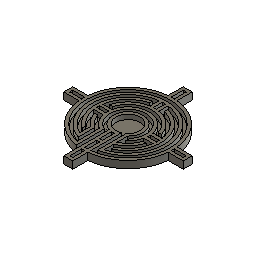
Labyrinth1 (5-gängig) v1 (Autodesk Fusion 360 design; units mm, degrees)
Autodesk Fusion 360 part; units mm, degrees
sketch "Skizze1" plane through (0, 0, 0) normal (0, 1, 0) x (1, 0, 0)
  circle A0 centre (0, 0) radius 15 construction
  circle A1 centre (0, 0) radius 20 construction
  circle A2 centre (0, 0) radius 25 construction
  circle A3 centre (0, 0) radius 30 construction
  circle A4 centre (0, 0) radius 35 construction
  line L0 (0, 0) -> (0, 68.1169) construction
  line L1 (0, 0) -> (0, -68.6498) construction
  line L2 (-1.25, 0) -> (-1.25, 68.1169) construction
  line L3 (-1.25, 0) -> (-1.25, -68.6498) construction
  line L4 (1.25, 0) -> (1.25, 68.1169) construction
  line L5 (1.25, 0) -> (1.25, -68.6498) construction
  line L6 (-3.75, 0) -> (-3.75, 68.1169) construction
  line L7 (-3.75, 0) -> (-3.75, -68.6498) construction
  line L8 (3.75, 0) -> (3.75, 68.1169) construction
  line L9 (3.75, 0) -> (3.75, -68.6498) construction
  line L10 (-6.25, 0) -> (-6.25, -68.6498) construction
  line L11 (-6.25, 0) -> (-6.25, 68.1169) construction
  line L12 (6.25, 0) -> (6.25, 68.1169) construction
  line L13 (6.25, 0) -> (6.25, -68.6498) construction
  line L14 (0, 0) -> (75.7523, 0) construction
  line L15 (0, 0) -> (-77.2035, 0) construction
  line L16 (0, -1.25) -> (-77.2035, -1.25) construction
  line L17 (0, -1.25) -> (75.7523, -1.25) construction
  line L18 (0, 1.25) -> (75.7523, 1.25) construction
  line L19 (0, 1.25) -> (-77.2035, 1.25) construction
  line L20 (0, 3.75) -> (75.7523, 3.75) construction
  line L21 (0, -3.75) -> (-77.2035, -3.75) construction
  line L22 (0, -3.75) -> (75.7523, -3.75) construction
  line L23 (0, -6.25) -> (75.7523, -6.25) construction
  line L24 (0, -6.25) -> (-77.2035, -6.25) construction
  line L25 (0, 6.25) -> (-77.2035, 6.25) construction
  line L26 (0, 6.25) -> (75.7523, 6.25) construction
  line L27 (0, 0) -> (50, 0) construction
  line L28 (0, 0) -> (-50, 0) construction
  line L29 (0, 0) -> (0, 50) construction
  line L30 (0, 0) -> (0, -50) construction
  line L31 (0, 50) -> (3.75, 50) construction
  line L32 (-50, 0) -> (-50, 3.75) construction
  line L33 (-50, 3.75) -> (50, 3.75) construction
  line L34 (50, 3.75) -> (50, -3.75) construction
  line L35 (50, -3.75) -> (-50, -3.75) construction
  line L36 (-50, -3.75) -> (-50, 3.75) construction
  line L37 (50, 3.75) -> (50, -3.75)
  line L38 (-50, -3.75) -> (-50, 3.75)
  line L39 (3.75, 50) -> (-3.75, 50)
  line L40 (-3.75, -50) -> (3.75, -50)
  circle A5 centre (0, 0) radius 12.5 construction
  arc A6 (6.25, -7.8334) -> (3.75, -9.2931) centre (0, 0) ccw
  line L41 (-6.25, -44.5639) -> (-6.25, -13.6359)
  line L42 (-6.25, 39.5087) -> (-6.25, 42.0379)
  circle A7 centre (0, 0) radius 37.5
  line L43 (-8.75, 0) -> (-8.75, -50) construction
  line L44 (-11.25, 0) -> (-11.25, -50) construction
  line L45 (11.25, 0) -> (11.25, -50) construction
  line L46 (8.75, 0) -> (8.75, -68.6498) construction
  line L47 (-1.25, -12.4373) -> (-1.25, -44.9826)
  line L48 (1.25, -12.4373) -> (1.25, -44.9826)
  arc A8 (-1.25, -12.4373) -> (1.25, -12.4373) centre (0, 0) ccw
  line L49 (3.75, -9.2931) -> (3.75, -42.3342)
  arc A9 (8.75, -8.9268) -> (-3.75, -11.9242) centre (0, 0) ccw
  line L50 (8.75, -39.0312) -> (8.7506, -41.5894)
  line L51 (-6.25, -44.5639) -> (-6.25, -49.6078)
  arc A10 (11.25, -9.9216) -> (-6.25, -13.6359) centre (0, 0) ccw
  arc A11 (11.25, -13.4048) -> (17.0935, -3.75) centre (0, 0) ccw
  arc A12 (8.75, -17.9844) -> (18.9984, -6.25) centre (0, 0) ccw
  line L52 (11.25, -9.9216) -> (11.25, -13.4048)
  arc A13 (8.75, -20.7289) -> (21.6145, -6.25) centre (0, 0) ccw
  line L53 (18.9984, -6.25) -> (21.6145, -6.25)
  arc A14 (11.25, -22.4692) -> (24.8468, -3.75) centre (0, 0) ccw
  arc A15 (11.25, -25.0936) -> (27.2431, -3.75) centre (0, 0) ccw
  line L54 (11.25, -22.4692) -> (11.25, -25.0936)
  arc A16 (27.2431, -3.75) -> (27.2431, 3.75) centre (0, 0) ccw
  arc A17 (27.2431, 3.75) -> (6.25, 26.7804) centre (0, 0) ccw
  arc A18 (24.7171, 3.75) -> (6.25, 24.2061) centre (0, 0) ccw
  line L55 (6.25, 26.7804) -> (6.25, 24.2061)
  arc A19 (8.75, -28.6956) -> (3.75, 29.7647) centre (0, 0) ccw
  arc A20 (6.25, -31.8934) -> (-11.25, -30.4908) centre (0, 0) ccw
  arc A21 (3.75, -34.7985) -> (-8.75, -33.8886) centre (0, 0) ccw
  arc A22 (17.0935, 3.75) -> (-8.75, -15.1554) centre (0, 0) ccw
  line L56 (-8.75, -15.1554) -> (-8.75, -33.8886)
  arc A23 (18.9984, 6.25) -> (3.75, 19.6453) centre (0, 0) ccw
  line L57 (3.75, 29.7647) -> (3.75, 19.6453)
  arc A24 (21.6145, 6.25) -> (3.75, 22.1853) centre (0, 0) ccw
  line L58 (18.9984, 6.25) -> (21.6145, 6.25)
  line L59 (3.75, 29.7647) -> (3.75, 32.2829)
  line L60 (-3.75, -11.9242) -> (-3.75, -50)
  arc A25 (3.75, -37.312) -> (-6.25, -36.9755) centre (0, 0) ccw
  line L61 (37.2821, 3.75) -> (50, 3.75)
  line L62 (50, 3.75) -> (50, -3.75)
  line L63 (50, -3.75) -> (37.312, -3.75)
  line L64 (-37.312, 3.75) -> (-50, 3.75)
  line L65 (-50, -3.75) -> (-37.312, -3.75)
  line L66 (-3.879, 37.2988) -> (-3.75, 50)
  line L67 (3.75, 50) -> (3.6612, 37.3208)
  arc A26 (3.75, 19.6453) -> (-18.9984, 6.25) centre (0, 0) ccw
  line L68 (6.25, -31.8934) -> (6.25, -7.8334)
  line L69 (8.75, -28.6956) -> (8.75, -20.7289)
  line L70 (8.75, -17.9844) -> (8.75, -8.9268)
  line L71 (-3.75, 32.2829) -> (-3.75, 19.6453)
  arc A27 (1.25, 22.4653) -> (-1.25, 22.4653) centre (0, 0) ccw
  arc A28 (1.25, 29.9739) -> (-1.25, 29.9739) centre (0, 0) ccw
  line L72 (1.25, 22.4653) -> (1.25, 29.9739)
  line L73 (-1.25, 22.4653) -> (-1.25, 29.9739)
  line L74 (17.0935, 3.75) -> (24.7171, 3.75)
  line L75 (17.0935, -3.75) -> (24.8468, -3.75)
  line L76 (3.75, -37.312) -> (3.75, -50)
  line L77 (-11.25, -16.5359) -> (-11.25, -30.4908)
  line L78 (-16.25, -16.5359) -> (-16.25, -30.4908) construction
  line L79 (-13.75, -16.5359) -> (-13.75, -30.4908) construction
  arc A29 (-18.9984, -6.25) -> (-11.25, -16.5359) centre (0, 0) ccw
  arc A30 (-21.6145, -6.25) -> (-13.75, -17.8098) centre (0, 0) ccw
  arc A31 (-6.25, 29.3417) -> (-13.75, -26.6634) centre (0, 0) ccw
  arc A32 (-6.25, 26.7804) -> (-26.7804, 6.25) centre (0, 0) ccw
  arc A33 (-3.75, 29.7647) -> (-6.25, 29.3417) centre (0, 0) ccw
  line L80 (-18.9984, -6.25) -> (-21.6145, -6.25)
  line L81 (-13.75, -17.8098) -> (-13.75, -26.6634)
  arc A34 (-26.7804, 6.25) -> (-16.25, -22.1853) centre (0, 0) ccw
  arc A35 (-6.25, 24.2061) -> (-24.7171, 3.75) centre (0, 0) ccw
  line L82 (-6.25, 26.7804) -> (-6.25, 24.2061)
  line L83 (-24.7171, 3.75) -> (-27.2431, 3.75)
  arc A36 (-24.791, -3.75) -> (-16.25, -19.0943) centre (0, 0) ccw
  line L84 (-16.25, -19.0943) -> (-16.25, -22.1853)
  line L85 (-24.791, -3.75) -> (-27.2431, -3.75)
  line L86 (-27.2431, 3.75) -> (-17.0935, 3.75)
  line L87 (-27.2431, -3.75) -> (-17.051, -3.75)
  arc A37 (-3.75, 22.1853) -> (-21.6145, 6.25) centre (0, 0) ccw
  line L88 (-21.6145, 6.25) -> (-18.9984, 6.25)
  line L89 (3.75, 47.5) -> (-3.75, 47.5) construction
  line L90 (-1.25, 47.5) -> (1.25, 47.5)
  line L91 (1.25, 47.5) -> (1.2613, 37.4788)
  line L92 (-1.299, 37.4775) -> (-1.25, 47.5)
  line L93 (-47.4997, -3.75) -> (-47.4997, 3.75) construction
  line L94 (47.4997, 3.75) -> (47.4997, -3.75) construction
  line L95 (-47.4997, -1.25) -> (-37.4792, -1.25)
  line L96 (-47.4997, 1.25) -> (-47.4997, -1.25)
  line L97 (-47.4997, 1.25) -> (-37.4792, 1.25)
  line L98 (47.4997, 1.25) -> (37.4792, 1.25)
  line L99 (47.4997, -1.25) -> (37.4792, -1.25)
  line L100 (47.4997, 1.25) -> (47.4997, -1.25)
  arc A38 (-24.9687, 1.25) -> (-24.9687, -1.25) centre (0, 0) ccw
  arc A39 (17.4553, -1.25) -> (17.4553, 1.25) centre (0, 0) ccw
  arc A40 (24.9687, -1.25) -> (24.9687, 1.25) centre (0, 0) ccw
  line L101 (17.4553, 1.25) -> (24.9687, 1.25)
  line L102 (17.4553, -1.25) -> (24.9687, -1.25)
  line L103 (-24.9687, 1.25) -> (-17.4553, 1.25)
  line L104 (-24.9687, -1.25) -> (-17.4553, -1.25)
  arc A41 (-1.25, -47.4835) -> (1.25, -47.4835) centre (0, 0) ccw
  line L105 (1.25, -37.4792) -> (1.25, -47.4835)
  line L106 (-1.25, -37.4567) -> (-1.25, -47.4835)
  arc A42 (-1.25, -24.9687) -> (1.25, -24.9687) centre (0, 0) ccw
  arc A43 (-1.25, -22.4653) -> (1.25, -22.4653) centre (0, 0) ccw
  arc A44 (-1.25, -34.8756) -> (1.25, -34.8756) centre (0, 0) ccw
  dimension "d9" = 1.25
  dimension "d10" = -1.25
  dimension "d11" = 3.75
  dimension "d12" = -3.75
  dimension "d13" = 6.25
  dimension "d15" = -6.25
  dimension "d16" = 1.25
  dimension "d17" = -1.25
  dimension "d19" = -3.75
  dimension "d20" = 6.25
  dimension "d21" = -6.25
  dimension "d22" = 50
  dimension "d23" = 50
  dimension "d24" = 50
  dimension "d25" = 50
  dimension "d44" = 37.5
  dimension "d46" = 5
  dimension "d47" = 2.5
  dimension "d48" = 22.5
  dimension "d50" = 22.5
  dimension "d51" = -2.5
  dimension "d52" = 2.5003
  dimension "d53" = 2.5003
  dimension "d54" = 17.5
  dimension "d59" = 47.5
  constraint coincident A0.centre A1.centre
  constraint concentric A0 A1
  constraint concentric A3 A4
  constraint vertical L0
  constraint vertical L1
  constraint horizontal L14
  constraint horizontal L15
  constraint parallel L14 L27
  constraint parallel L16 L28
  constraint parallel L0 L29
  constraint parallel L1 L30
  constraint coincident L8 L31.end
  constraint perpendicular L8 L31
  constraint horizontal L33
  constraint vertical L34
  constraint horizontal L35
  constraint vertical L36
  constraint coincident L22 L34.end
  constraint vertical L37
  constraint vertical L38
  constraint horizontal L39
  constraint horizontal L40
  constraint coincident L7 L40.start
  constraint concentric A1 A5
  constraint coincident L13 A6.start
  constraint coincident L9 A6.end
  constraint coincident L10 L41.start
  constraint coincident L10 L41.end
  constraint coincident A0 L41.end
  constraint coincident L11 L42.start
  constraint coincident L11 L42.end
  constraint coincident L3 L47.start
  constraint coincident A5 L47.start
  constraint coincident L3 L47.end
  constraint coincident A5 L48.start
  constraint coincident L5 L48.start
  constraint coincident L5 L48.end
  constraint coincident L9 L49.end
  constraint coincident L7 A9.end
  constraint coincident A5 A9.start
  constraint coincident L46 A9.start
  constraint coincident L46 L50.start
  constraint coincident L10 L51.end
  constraint coincident L45 A10.start
  constraint coincident L22 A11.end
  constraint coincident L45 A11.start
  constraint coincident L23 A12.end
  constraint coincident A1 A12.start
  constraint coincident L46 A13.start
  constraint coincident L23 A13.end
  constraint coincident L45 A14.start
  constraint coincident L22 A14.end
  constraint coincident L45 A15.start
  constraint coincident L22 A15.end
  constraint coincident L12 A17.end
  constraint coincident L20 A18.start
  constraint coincident L12 A18.end
  constraint coincident A2 A18.end
  constraint coincident L8 A19.end
  constraint coincident L46 A19.start
  constraint coincident L44 A20.end
  constraint coincident L43 A21.end
  constraint coincident A4 A21.start
  constraint coincident L9 A21.start
  constraint coincident L20 A22.start
  constraint coincident L43 A22.end
  constraint coincident L8 A23.end
  constraint coincident L26 A23.start
  constraint coincident A1 A23.start
  constraint coincident L8 A24.end
  constraint coincident L26 A24.start
  constraint coincident L8 L59.end
  constraint coincident A20 L59.end
  constraint coincident L10 A25.end
  constraint coincident L33 L61.start
  constraint perpendicular L34 L61
  constraint coincident L35 L63.end
  constraint coincident A7 L63.end
  constraint coincident L33 L64.start
  constraint coincident A7 L64.start
  constraint perpendicular L32 L64
  constraint coincident L21 L65.end
  constraint coincident A7 L65.end
  constraint coincident A7 L66.start
  constraint coincident A25 L66.start
  constraint coincident A25 L67.end
  constraint coincident A7 L67.end
  constraint coincident L25 A26.end
  constraint parallel L13 L68
  constraint parallel L46 L70
  constraint coincident L6 L71.start
  constraint coincident A20 L71.start
  constraint coincident L6 L71.end
  constraint coincident A26 L71.end
  constraint coincident A1 L71.end
  constraint coincident L2 A27.end
  constraint coincident L4 A27.start
  constraint coincident L2 A28.end
  constraint coincident A3 A28.start
  constraint coincident L4 A28.start
  constraint perpendicular L40 L76
  constraint coincident A1 L77.start
  constraint coincident L44 L77.start
  constraint coincident L24 A29.start
  constraint coincident L79 A30.end
  constraint coincident L24 A30.start
  constraint coincident L11 A31.start
  constraint coincident L79 A31.end
  constraint coincident A3 A31.end
  constraint coincident L25 A32.end
  constraint coincident L11 A32.start
  constraint coincident L6 A33.start
  constraint coincident L78 A34.end
  constraint coincident L35 A36.start
  constraint coincident L33 A35.end
  constraint coincident A2 A35.end
  constraint coincident L11 A35.start
  constraint coincident L33 L83.end
  constraint coincident A34 L83.end
  constraint coincident L78 A36.end
  constraint coincident L21 L85.end
  constraint coincident A34 L85.end
  constraint coincident L33 L86.end
  constraint coincident A22 L86.end
  constraint coincident L21 L87.end
  constraint coincident L25 A37.end
  constraint coincident L6 A37.start
  constraint coincident L89 L90.start
  constraint coincident L2 L90.start
  constraint coincident L4 L90.end
  constraint coincident L89 L90.end
  constraint midpoint A25 L91.end
  constraint coincident A7 L92.start
  constraint coincident A25 L92.start
  constraint coincident L19 L96.start
  constraint coincident L93 L96.start
  constraint coincident L16 L95.start
  constraint coincident L93 L95.start
  constraint coincident L16 L95.end
  constraint coincident A7 L95.end
  constraint coincident A25 L95.end
  constraint coincident L19 L97.end
  constraint coincident A25 L97.end
  constraint coincident A7 L97.end
  constraint coincident L94 L98.start
  constraint coincident L18 L98.start
  constraint coincident A7 L98.end
  constraint coincident L18 L98.end
  constraint coincident A25 L98.end
  constraint coincident L94 L99.start
  constraint coincident L17 L99.start
  constraint coincident L17 L99.end
  constraint coincident A7 L99.end
  constraint coincident L16 A38.end
  constraint coincident L19 A38.start
  constraint coincident A2 A38.start
  constraint coincident L18 A39.end
  constraint coincident L17 A39.start
  constraint coincident L17 A40.start
  constraint coincident L18 A40.end
  constraint coincident A2 A40.end
  constraint coincident L19 L103.end
  constraint coincident A22 L103.end
  constraint coincident A22 L104.end
  constraint coincident L16 L104.end
  constraint coincident L3 A41.start
  constraint coincident L5 A41.end
  constraint coincident L48 L105.start
  constraint coincident A7 L105.start
  constraint coincident L47 L106.start
  constraint coincident L3 A42.start
  constraint coincident A2 A42.end
  constraint coincident L48 A42.end
  constraint coincident L3 A43.start
  constraint coincident L48 A43.end
  constraint coincident L3 A44.start
  constraint coincident L48 A44.end
  measures "d22" distance of A0.centre L27.end
  measures "d23" distance of A0.centre L28.end
  measures "d24" distance of A0.centre L29.end
  measures "d25" distance of A0.centre L30.end
  measures "d44" radius of A25
  measures "d48" radius of A30
  measures "d50" radius of A37
  measures "d54" radius of A39
  measures "d59" radius of A41
extrude "Extrusion3" add sketch "Skizze1" against normal blind 2 contours L37 A7 A25 L61 L62 L63 L98 L99 L100 | L41 A7 L49 A10 A11 L52 A14 A15 L54 A16 A17 A18 L55 A21 A22 L56 A25 L74 L75 | A7 A25 L98 L99 L100 | L39 A7 A25 L66 L67 L90 L91 L92 | L40 A7 L47 L48 L49 L60 L76 A41 L105 L106 | A6 A7 L47 L48 A8 L49 A9 A12 A13 L53 A19 A20 L59 L60 L68 L69 L70 L106 | A7 A25 L90 L91 L92 | A7 L47 L48 A41 L105 L106 | A7 L47 L48 L106 A44 | A6 L41 A7 L49 A9 A10 A11 A12 L52 A13 L53 A14 A15 L54 A16 A17 A18 L55 A19 A20 A21 A22 L56 A23 L57 A24 L58 L60 A26 L68 L69 L70 L71 L74 L75 L77 A29 A30 A31 A32 A33 L80 L81 A34 A35 L82 A36 L84 L86 L87 A37 L88 | L47 L48 A42 A44 | L47 L48 A42 A43 | L38 A7 A25 L64 L65 L95 L96 L97 | L47 L48 A8 A43 | A22 A34 L83 L85 L86 L87 A38 L103 L104 | A7 A25 L95 L96 L97 | A20 L57 L59 A26 L71 | A22 A38 L103 L104 | A34 A36 L84 L85 L87 | A20 L71 L77 A29 A30 A31 A33 L80 L81 | A23 L57 A24 L58 | A32 A34 A35 L82 L83 L86 | A26 L71 A37 L88 | A27 A28 L72 L73 | A39 A40 L101 L102
extrude "Extrusion5" add sketch "Skizze1" along normal blind 4 contours L37 A7 A25 L61 L62 L63 L98 L99 L100 | L41 A7 L49 A10 A11 L52 A14 A15 L54 A16 A17 A18 L55 A21 A22 L56 A25 L74 L75 | L39 A7 A25 L66 L67 L90 L91 L92 | L40 A7 L47 L48 L49 L60 L76 A41 L105 L106 | A6 A7 L47 L48 A8 L49 A9 A12 A13 L53 A19 A20 L59 L60 L68 L69 L70 L106 | A7 L47 L48 L106 A44 | L47 L48 A42 A43 | L38 A7 A25 L64 L65 L95 L96 L97 | A22 A34 L83 L85 L86 L87 A38 L103 L104 | A20 L57 L59 A26 L71 | A34 A36 L84 L85 L87 | A20 L71 L77 A29 A30 A31 A33 L80 L81 | A23 L57 A24 L58 | A32 A34 A35 L82 L83 L86 | A26 L71 A37 L88
equation "d11 = 0.125 cm + 0.25 cm"
equation "d12 = -0.125 cm - 0.25 cm"
equation "d13 = 0.125 cm + 0.5 cm"
equation "d15 = -0.125 cm - 0.5 cm"
equation "d19 = -0.125 cm - 0.25 cm"
equation "d20 = 0.125 cm + 0.5 cm"
equation "d21 = -0.125 cm - 0.5 cm"
named bodies: "Boden"
